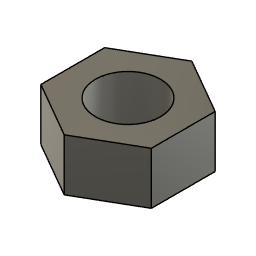
M10 nut v1 (Autodesk Fusion 360 design; units mm, degrees)
Autodesk Fusion 360 part; units mm, degrees
sketch "Sketch1" plane through (0, 0, 0) normal (0, 1, 0) x (1, 0, 0)
  circle A0 centre (0, 0) radius 5
  line L0 (-8.5, -4.9075) -> (0, -9.815)
  line L1 (0, -9.815) -> (8.5, -4.9075)
  line L2 (8.5, -4.9075) -> (8.5, 4.9075)
  line L3 (8.5, 4.9075) -> (0, 9.815)
  line L4 (0, 9.815) -> (-8.5, 4.9075)
  line L5 (-8.5, 4.9075) -> (-8.5, -4.9075)
  dimension "d1" = 10
  dimension "d3" = 17
  constraint coincident A0.centre origin
  constraint vertical L5
  measures "d1" diameter of A0
  measures "d3" distance of L2 L5
extrude "Extrude1" add sketch "Sketch1" along normal blind 8 makes body 1
copy_body "Body->Comp1" bodies 1 removing the originals makes body 2 in component "M10 nut"
component "M10 nut" placed x (1, 0, 0) y (0, 1, 0) z (0, 0, 1) at (0, 0, 0)
named bodies: "M10 nut"
